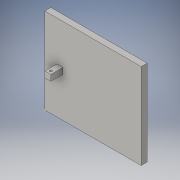
# Autodesk Inventor part: HingePart1MK2
Saved by Autodesk Inventor 2016 (Build 200138000, 138)
## iProperties
Created: 2017-02-18
Part Number: HingePart1MK2
Material: Generic
Document SubType Name: Modeling
Designer: RoboticsUser
Density: 1 g/cm^3
Appearance: Default
Author: RoboticsUser
Autodesk Inventor part; units mm, degrees
ref_plane "YZ Plane" through (0, 0, 0) normal (1, 0, 0) x (0, 1, 0)
ref_plane "XZ Plane" through (0, 0, 0) normal (0, 1, 0) x (-1, 0, 0)
ref_plane "XY Plane" through (0, 0, 0) normal (0, 0, 1) x (1, 0, 0)
sketch "Sketch1" plane through (0, 0, 0) normal (0, 0, 1) x (1, 0, 0)
  line L0 (0, 0) -> (50.8, 0)
  line L1 (50.8, 0) -> (50.8, 45.212)
  line L2 (50.8, 45.212) -> (0, 45.212)
  line L3 (0, 45.212) -> (0, 0)
  dimension "d0" = 50.8
  dimension "d1" = 45.212
  constraints: 8 end point, 2 parallel, 1 horizontal, 1 perpendicular
  measures "d0" distance of L2.end L1.end
  measures "d1" distance of L1.end L0.end
extrude "Extrusion1" add sketch "Sketch1" along normal blind 3.175
sketch "Sketch3" plane through (0, 0, 3.175) normal (0, 0, 1) x (1, 0, 0)
  point P0 (0, 0)
sketch "Sketch4" plane through (0, 0, 3.175) normal (0, 0, 1) x (1, 0, 0)
  point P0 (0, 0)
sketch "Sketch5" plane through (0, 0, 3.175) normal (0, 0, 1) x (1, 0, 0)
  line L0 (6.35, 21.0058) -> (9.525, 21.0058)
  line L1 (9.525, 21.0058) -> (9.525, 24.1808)
  line L2 (9.525, 24.1808) -> (6.35, 24.1808)
  line L3 (6.35, 24.1808) -> (6.35, 21.0058)
  point P0 (0, 0)
  dimension "d12" = 3.175
  dimension "d13" = 3.175
  constraints: 8 end point, 2 parallel, 1 horizontal, 1 perpendicular
  measures "d12" distance of L2.end L1.end
  measures "d13" distance of L1.end L0.end
extrude "Extrusion3" add sketch "Sketch5" along normal blind 6.35
hole "Hole1" at (7.9248, 21.0058, 7.9248) direction (0, 1, 0) diameter 1.27 end through all
body "Solid1"
